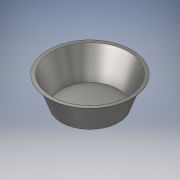
# Autodesk Inventor part: bowl-2
Saved by Autodesk Inventor 2018 (Build 220112000, 112)
## iProperties
Created: 2018-03-29
Part Number: bowl-2
Material: Stainless Steel
Document SubType Name: Modeling
Designer: guita
Density: 8 g/cm^3
Appearance: Semi-Polished
Author: guita
Autodesk Inventor part; units mm, degrees
ref_plane "YZ Plane" through (0, 0, 0) normal (1, 0, 0) x (0, 1, 0)
ref_plane "XZ Plane" through (0, 0, 0) normal (0, 1, 0) x (-1, 0, 0)
ref_plane "XY Plane" through (0, 0, 0) normal (0, 0, 1) x (1, 0, 0)
sketch "Sketch1" plane through (0, 0, 0) normal (1, 0, 0) x (0, 1, 0)
  line L0 (0, 0) -> (0, -38.1)
  line L1 (0, 0) -> (36.5125, 0)
  line L2 (36.5125, -51.0466) -> (36.5125, -57.15)
  line L3 (36.5125, -57.15) -> (35.1989, -57.15)
  line L4 (34.925, -50.8) -> (0, -38.1)
  line L5 (36.5125, -55.5625) -> (36.5125, -57.15)
  line L6 (36.5125, -55.5625) -> (36.1823, -55.5625)
  line L7 (36.1823, -55.5625) -> (36.1823, -51.2572)
  line L8 (36.1823, -55.5625) -> (40.5858, -55.5625) construction
  line L9 (34.925, -50.8) -> (36.1823, -51.2572)
  arc A0 (36.516, -55.6063) -> (36.5125, -55.5625) centre (35.0619, -55.6994) ccw
  line L10 (35.1989, -57.15) -> (36.1823, -55.5625)
  line L11 (0, 0) -> (0.3302, 0)
  line L12 (0.3302, 0) -> (0.1665, -37.8298)
  line L13 (36.1837, -50.927) -> (0.1665, -37.8298)
  line L14 (36.1837, -50.927) -> (36.5125, -51.0466)
  dimension "d0" = 38.1
  dimension "d1" = 36.5125
  dimension "d2" = 57.15
  dimension "d5" = 0.3302
  dimension "d6" = 90
  dimension "d7" = 0.3302
  constraints: 30 end point, 3 horizontal, 2 perpendicular, 2 point on circle, 2 point on line, 1 centre point, 1 parallel, 1 vertical
  measures "d0" distance of L0.start L0.end
  measures "d1" distance of L0.start L1.end
  measures "d2" distance of L1.end L2.end
  measures "d5" distance of L5.start L6.end
  measures "d6" angle of L8 L7
  measures "d7" distance of L0.start L11.end
revolve "Revolution1" add sketch "Sketch1" angle 360 about axis through (0, 0, 0) along (0, 1, 0) contours L1 L12 L13 L14 L2 L6 L7 L9 L4 L0
body "Solid1"
